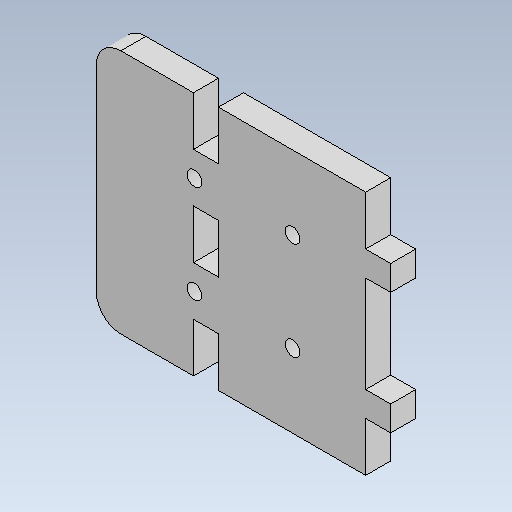
# Autodesk Inventor part: motor chasis holder
Saved by Autodesk Inventor 2025 (Build 290162000, 162)
## iProperties
Created: 2024-08-13
Part Number: motor chasis holder
Material: Polycarbonate, Smoke
Document SubType Name: Modeling
Designer: PC
Density: 1.2 g/cm^3
Appearance: Default
Author: PC
Autodesk Inventor part; units mm, degrees
ref_plane "YZ Plane" through (0, 0, 0) normal (1, 0, 0) x (0, 1, 0)
ref_plane "XZ Plane" through (0, 0, 0) normal (0, 1, 0) x (-1, 0, 0)
ref_plane "XY Plane" through (0, 0, 0) normal (0, 0, 1) x (1, 0, 0)
sketch "Sketch1" plane through (0, 0, 0) normal (0, 0, 1) x (1, 0, 0)
  line L0 (30, -25) -> (-25, -25)
  line L1 (-30, -20) -> (-30, 20)
  line L2 (-25, 25) -> (30, 25)
  line L3 (30, 25) -> (30, -25)
  line L4 (30, -25) -> (-30, 25) construction
  line L5 (-30, -25) -> (30, 25) construction
  circle A0 centre (-10, 10) radius 1.5
  circle A1 centre (-10, -10) radius 1.5
  circle A2 centre (10, 10) radius 1.5
  circle A3 centre (10, -10) radius 1.5
  arc A4 (-25, 25) -> (-30, 20) centre (-25, 20) ccw
  arc A5 (-30, -20) -> (-25, -25) centre (-25, -20) ccw
  point P0 (0, 0)
  dimension "d0" = 60
  dimension "d1" = 50
  dimension "d2" = 3
  dimension "d3" = 3
  dimension "d4" = 3
  dimension "d5" = 3
  dimension "d6" = 10
  dimension "d7" = 10
  dimension "d8" = 10
  dimension "d9" = 10
  dimension "d10" = 10
  dimension "d11" = 10
  dimension "d12" = 10
  dimension "d13" = 10
  dimension "d14" = 5
  constraints: 12 end point, 6 centre point, 4 point on circle, 4 point on line, 4 tangent, 2 midpoint, 2 parallel, 1 equal radius, 1 horizontal, 1 perpendicular
  measures "d0" distance of L4.end L2.end
  measures "d1" distance of L5.start L4.end
  measures "d2" diameter of A0
  measures "d3" diameter of A1
  measures "d4" diameter of A2
  measures "d5" diameter of A3
  measures "d6" horizontal distance of point (0, 0) A0.centre
  measures "d7" horizontal distance of point (0, 0) A1.centre
  measures "d8" horizontal distance of point (0, 0) A2.centre
  measures "d9" horizontal distance of point (0, 0) A3.centre
  measures "d10" horizontal distance of point (0, 0) A0.centre
  measures "d11" horizontal distance of point (0, 0) A2.centre
  measures "d12" horizontal distance of point (0, 0) A3.centre
  measures "d13" horizontal distance of A1.centre point (0, 0)
  measures "d14" radius of A4
extrude "Extrusion1" add sketch "Sketch1" along normal blind 5.1
sketch "Sketch4" plane through (0, 0, 0) normal (0, 0, -1) x (-1, 0, 0)
  line L0 (-30, 25) -> (25, 25) projected
  line L1 (-30, 25) -> (-24.9, 25)
  line L2 (-24.9, 25) -> (-24.9, 14.95)
  line L3 (-24.9, 14.95) -> (-30, 14.95)
  line L4 (-30, 14.95) -> (-30, 25)
  line L5 (-30, -25) -> (-30, 25) projected
  line L6 (-30, 9.85) -> (-24.9, 9.85)
  line L7 (-24.9, 9.85) -> (-24.9, -9.85)
  line L8 (-24.9, -9.85) -> (-30, -9.85)
  line L9 (-30, -9.85) -> (-30, 9.85)
  line L10 (25, -25) -> (-30, -25) projected
  line L11 (-30, -25) -> (-24.9, -25)
  line L12 (-24.9, -25) -> (-24.9, -14.95)
  line L13 (-24.9, -14.95) -> (-30, -14.95)
  line L14 (-30, -14.95) -> (-30, -25)
  point P0 (0, 0)
  point P1 (-24.9, 0)
  point P2 (-30, 0)
  dimension "d27" = 5.1
  dimension "d28" = 10.05
  dimension "d29" = 5.1
  dimension "d30" = 19.7
  dimension "d31" = 10.05
  dimension "d32" = 5.1
  constraints: 24 end point, 6 parallel, 3 horizontal, 3 perpendicular, 2 midpoint, 1 horizontal alignment, 1 point on line
  measures "d27" distance of L2.end L3.end
  measures "d28" distance of L1.end L2.end
  measures "d29" distance of L7.end L8.end
  measures "d30" distance of L6.end L7.end
  measures "d31" distance of L12.end L11.end
  measures "d32" distance between parallel lines of L5 L12
extrude "Extrusion5" cut sketch "Sketch4" against normal blind 40
sketch "Sketch5" plane through (0, 0, 5.1) normal (0, 0, 1) x (1, 0, 0)
  circle A0 centre (10, -10) radius 1.5 projected
  circle A1 centre (10, 10) radius 1.5 projected
  line L0 (24.9, -25) -> (24.9, -14.95) projected
  line L1 (24.9, -14.95) -> (30, -14.95) projected
  line L2 (30, -14.95) -> (30, -9.85) projected
  line L3 (30, -9.85) -> (24.9, -9.85) projected
  line L4 (24.9, -9.85) -> (24.9, 9.85) projected
  line L5 (24.9, 9.85) -> (30, 9.85) projected
  line L6 (30, 9.85) -> (30, 14.95) projected
  line L7 (30, 14.95) -> (24.9, 14.95) projected
  line L8 (24.9, 14.95) -> (24.9, 25) projected
  line L9 (24.9, 25) -> (-25, 25) projected
  arc A2 (-25, 25) -> (-30, 20) centre (-25, 20) ccw projected
  line L10 (-30, 20) -> (-30, -20) projected
  arc A3 (-30, -20) -> (-25, -25) centre (-25, -20) ccw projected
  line L11 (-25, -25) -> (24.9, -25) projected
  line L12 (-10.2, 5) -> (-5.1, 5)
  line L13 (-5.1, 5) -> (-5.1, -5)
  line L14 (-5.1, -5) -> (-10.2, -5)
  line L15 (-10.2, -5) -> (-10.2, 5)
  line L16 (-10.2, -15) -> (-5.1, -15)
  line L17 (-5.1, -15) -> (-5.1, -25)
  line L18 (-5.1, -25) -> (-10.2, -25)
  line L19 (-10.2, -25) -> (-10.2, -15)
  line L20 (-10.2, 15) -> (-5.1, 15)
  line L21 (-5.1, 15) -> (-5.1, 25)
  line L22 (-5.1, 25) -> (-10.2, 25)
  line L23 (-10.2, 25) -> (-10.2, 15)
  line L24 (-43.2426, 0) -> (42.2071, 0) construction
  point P0 (0, 0)
  dimension "d35" = 5.1
  dimension "d36" = 5.1
  dimension "d37" = 5.1
  dimension "d38" = 19.7
  dimension "d40" = 30
  dimension "d43" = 10
  dimension "d44" = 10
  constraints: 24 end point, 6 parallel, 3 horizontal, 3 perpendicular, 2 collinear, 1 point on line, 3 other
  measures "d35" distance between parallel lines of L21 L23
  measures "d36" distance between parallel lines of L13 L15
  measures "d37" distance between parallel lines of L17 L19
  measures "d38" distance between parallel lines of L3 L5
  measures "d40" distance between parallel lines of L4 L13
  measures "d43" distance between parallel lines of L12 L20
  measures "d44" distance between parallel lines of L14 L12
extrude "Extrusion6" cut sketch "Sketch5" against normal through all contours L11 L19 L16 L17 | L9 L21 L20 L23 | L12 L13 L14 L15
equation "\"d36\" = d35"
equation "\"d37\" = d36"
equation "\"d44\" = d43"
body "Solid1"
